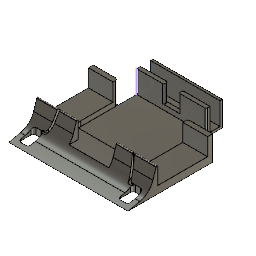
RASCUNHO_CHASSI (Autodesk Fusion 360 design; units mm, degrees)
Autodesk Fusion 360 part; units mm, degrees
sketch "Esboço1" plane through (0, 0, 0) normal (0, 0, 1) x (1, 0, 0)
  line L0 (0, 0) -> (240, 0)
  line L1 (0, 0) -> (0, 170)
  line L2 (0, 170) -> (50, 170)
  line L3 (50, 170) -> (50, 240)
  line L4 (190, 240) -> (190, 170)
  line L5 (190, 170) -> (240, 170)
  line L6 (240, 170) -> (240, 0)
  line L7 (50, 240) -> (190, 240)
  line L8 (10, 10) -> (10, 40)
  line L9 (30, 10) -> (30, 40)
  line L10 (30, 40) -> (10, 40)
  line L11 (10, 10) -> (30, 10)
  line L12 (230, 10) -> (210, 10)
  line L13 (210, 40) -> (230, 40)
  line L14 (210, 40) -> (210, 10)
  line L15 (230, 40) -> (230, 10)
  dimension "d2" = 170
  dimension "d3" = 170
  dimension "d4" = 240
  dimension "d6" = 50
  dimension "d8" = 140
  dimension "d9" = 70
  constraint coincident L0.start L1.start
  constraint horizontal L0
  constraint perpendicular L0 L1
  constraint perpendicular L1 L2
  constraint perpendicular L2 L3
  constraint perpendicular L2 L4
  constraint perpendicular L4 L5
  constraint perpendicular L2 L6
  constraint perpendicular L4 L7
  constraint perpendicular L0 L8
  constraint perpendicular L0 L9
  constraint perpendicular L9 L10
  constraint perpendicular L9 L11
  constraint perpendicular L6 L12
  constraint perpendicular L6 L13
  constraint perpendicular L12 L14
  constraint perpendicular L12 L15
  measures "d2" distance of L5.end L0.end
  measures "d3" distance of L0.start L1.end
  measures "d4" distance of L0.start L0.end
  measures "d6" distance of L4.end L5.end
  measures "d8" distance of L3.end L4.start
  measures "d9" distance of L2.end L3.end
extrude "Extrusão1" add sketch "Esboço1" along normal blind 15
fillet "Arredondamento2" radius 495 1 edges at (120, 0, 15)
sketch "Esboço5" plane through (0, 0, 0) normal (1, 0, 0) x (0, 1, 0)
  line L0 (43.5411, 8.5369) -> (60, 60)
  line L1 (60, 60) -> (60, 11)
  line L2 (43.5411, 8.5369) -> (60, 11)
  constraint vertical L1
extrude "Extrusão4" add sketch "Esboço5" along normal blind 240
fillet "Arredondamento3" radius 1.85 1 edges at (120, 60, 60)
fillet "Arredondamento4" radius 35 1 edges at (120, 43.6676, 8.9324)
delete_face "DeleteFace1" 1 faces at (80, 66.7415, 12.0246)
sketch "Esboço7" plane through (0, 0, 15) normal (0, 0, 1) x (-1, 0, 0)
  line L0 (0, -170) -> (0, -60)
  line L1 (0, -60) -> (-240, -60)
  line L2 (-240, -60) -> (-240, -170)
  line L3 (-240, -170) -> (-190, -170)
  line L4 (-190, -170) -> (-190, -240)
  line L5 (-190, -240) -> (-50, -240)
  line L6 (-50, -240) -> (-50, -170)
  line L7 (-50, -170) -> (0, -170)
  line L8 (-190, -170) -> (-190, -80)
  line L9 (-178.6152, -90) -> (-178.6152, -80)
  line L10 (-190, -80) -> (-50, -80)
  line L11 (-50, -80) -> (-50, -170)
  line L12 (-190, -170) -> (-190, -180)
  line L13 (-50, -170) -> (-50, -185)
  line L14 (-190, -185) -> (-50, -185)
  line L15 (-190, -185) -> (-190, -170)
  line L16 (-190, -170) -> (-190, -185)
  dimension "d34" = 140
  constraint coincident L3.end L4.start
  constraint perpendicular L3 L8
  constraint perpendicular L7 L9
  constraint perpendicular L8 L10
  constraint coincident L6.end L7.start
  constraint perpendicular L7 L11
  constraint coincident L4 L12.end
  constraint coincident L6 L13.end
  constraint perpendicular L7 L13
  constraint coincident L4 L14.start
  constraint perpendicular L6 L14
  measures "d34" distance of L8.end L10.end
extrude "Extrusão5" cut sketch "Esboço7" against normal blind 10 contours L4 L6 L8 L10 L11 L12 L13 L14 L15 L16
fillet "Arredondamento5" radius 15 1 edges at (190, 80, 10)
fillet "Arredondamento6" radius 15 1 edges at (50, 80, 10)
fillet "Arredondamento7" radius 5 1 edges at (230, 40, 6.7494)
fillet "Arredondamento8" radius 5 1 edges at (210, 40, 6.7494)
fillet "Arredondamento9" radius 5 1 edges at (10, 40, 6.7494)
fillet "Arredondamento10" radius 5 1 edges at (30, 40, 6.7494)
fillet "Arredondamento11" radius 5 1 edges at (10, 10, 1.2046)
fillet "Arredondamento12" radius 5 1 edges at (30, 10, 1.2046)
fillet "Arredondamento13" radius 5 1 edges at (230, 10, 1.2046)
fillet "Arredondamento14" radius 5 1 edges at (210, 10, 1.2046)
sketch "Esboço9" plane through (0, 0, 0) normal (0, 1, 0) x (1, 0, 0)
  line L0 (160, -50) -> (80, -50)
  line L1 (160, -50) -> (240, -50)
  line L2 (80, -50) -> (0, -50)
  line L3 (160, -50) -> (160, -15)
  line L4 (160, -15) -> (80, -15)
  line L5 (80, -15) -> (80, -50)
  dimension "d59" = 80
  constraint horizontal L0
  constraint parallel L0 L1
  constraint parallel L0 L2
  constraint equal L1 L2
  constraint equal L0 L2
  constraint perpendicular L0 L3
  constraint perpendicular L3 L4
  constraint perpendicular L0 L5
  measures "d59" distance of L0.start L0.end
extrude "Extrusão6" cut sketch "Esboço9" along normal blind 70
extrude "Extrusão7" cut 1 faces at (96.6667, 203.3333, 15) along direction (0, 0, -1) blind 10
sketch "Esboço10" plane through (0, 0, 5) normal (0, 0, 1) x (-1, 0, 0)
  arc A0 (-50, -95) -> (-65, -80) centre (-65, -95) ccw
  line L0 (-65, -80) -> (-175, -80)
  arc A1 (-175, -80) -> (-190, -95) centre (-175, -95) ccw
  line L1 (-190, -95) -> (-190, -170)
  line L2 (-190, -170) -> (-190, -240)
  line L3 (-190, -240) -> (-50, -240)
  line L4 (-50, -240) -> (-50, -170)
  line L5 (-50, -170) -> (-50, -95)
  line L6 (-190, -240) -> (-50, -240)
  line L7 (-190, -240) -> (-190, -235)
  line L8 (-50, -235) -> (-190, -235)
  line L9 (-50, -240) -> (-50, -235)
  constraint coincident L2.end L3.start
  constraint coincident L3.end L4.start
  constraint coincident L2 L7.end
  constraint perpendicular L3 L7
  constraint coincident L4 L8.start
  constraint perpendicular L2 L8
extrude "Extrusão8" add sketch "Esboço10" along normal blind 40 contours L2 L3 L4 L6 L7 L8 L9
sketch "Esboço15" plane through (0, 0, 0) normal (1, 0, 0) x (0, 1, 0)
extrude "Extrusão9" add 1 faces at (143.3333, 238.3333, 45) along direction (0, 0, 1) blind 5
sketch "Esboço17" plane through (0, 0, 5) normal (0, 0, 1) x (-1, 0, 0)
  line L0 (-190, -235) -> (-50, -235)
  line L1 (-50, -235) -> (-50, -170)
  line L2 (-50, -170) -> (-50, -95)
  arc A0 (-50, -95) -> (-65, -80) centre (-65, -95) ccw
  line L3 (-65, -80) -> (-175, -80)
  arc A1 (-175, -80) -> (-190, -95) centre (-175, -95) ccw
  line L4 (-190, -95) -> (-190, -170)
  line L5 (-190, -170) -> (-190, -235)
  line L6 (-50, -215) -> (-190, -215)
  line L7 (-190, -210) -> (-190, -215)
  line L8 (-50, -215) -> (-50, -210)
  line L9 (-190, -210) -> (-190, -207.0502)
  line L10 (-50, -207.0502) -> (-50, -210)
  line L11 (-190, -207.0502) -> (-50, -207.0502)
  constraint coincident L1 L6.start
  constraint perpendicular L1 L6
  constraint coincident L5 L7.start
  constraint perpendicular L6 L7
  constraint coincident L1 L8.end
  constraint coincident L5 L9.end
  constraint parallel L5 L9
  constraint coincident L1 L10.start
  constraint perpendicular L1 L11
extrude "Extrusão10" add sketch "Esboço17" along normal blind 45 contours L1 L5 L6 L7 L8 L9 L10 L11
sketch "Esboço18" plane through (50, 0, 0) normal (-1, 0, 0) x (0, -1, 0)
  line L0 (-170, 5) -> (-207.0502, 5)
  line L1 (-207.0502, 50) -> (-215, 50)
  line L2 (-215, 50) -> (-215, 5)
  line L3 (-215, 5) -> (-235, 5)
  line L4 (-235, 5) -> (-235, 50)
  line L5 (-235, 50) -> (-240, 50)
  line L6 (-240, 50) -> (-240, 0)
  line L7 (-240, 0) -> (-170, 0)
  line L8 (-170, 0) -> (-170, 5)
  line L9 (-207.0502, 5) -> (-207.0502, 50)
sketch "Esboço20" plane through (0, 0, 50) normal (0, 0, 1) x (-1, 0, 0)
  line L0 (-50, -207.0502) -> (-190, -207.0502)
  line L1 (-190, -207.0502) -> (-190, -215)
  line L2 (-190, -215) -> (-50, -215)
  line L3 (-50, -215) -> (-50, -207.0502)
  line L4 (-135.1601, -207.0502) -> (-105, -207.0502)
  line L5 (-135.1601, -207.0502) -> (-135, -215)
  line L6 (-105, -207.0502) -> (-105, -215)
  line L7 (-135, -215) -> (-105, -215)
  constraint coincident L0 L4.start
  constraint coincident L0 L4.end
  constraint coincident L2 L5.end
  constraint coincident L2 L6.end
  constraint perpendicular L6 L7
extrude "Extrusão11" cut sketch "Esboço20" against normal blind 35 contours L0 L2 L4 L5 L6 L7
sketch "Esboço22" plane through (0, 0, 15) normal (0, 0, 1) x (-1, 0, 0)
  line L0 (-160, -60) -> (-240, -60)
  line L1 (-240, -60) -> (-240, -170)
  line L2 (-240, -170) -> (-190, -170)
  line L3 (-190, -170) -> (-190, -95)
  arc A0 (-175, -80) -> (-190, -95) centre (-175, -95) ccw
  line L4 (-175, -80) -> (-65, -80)
  arc A1 (-50, -95) -> (-65, -80) centre (-65, -95) ccw
  line L5 (-50, -95) -> (-50, -170)
  line L6 (-50, -170) -> (0, -170)
  line L7 (0, -170) -> (0, -60)
  line L8 (0, -60) -> (-80, -60)
  line L9 (-80, -60) -> (-80, -41.5864)
  line L10 (-80, -41.5864) -> (-160, -41.5864)
  line L11 (-160, -41.5864) -> (-160, -60)
  line L12 (-240, -170) -> (-240, -160)
  line L13 (-190, -160) -> (-190, -170)
  line L14 (-240, -160) -> (-190, -160)
  line L15 (-50, -160) -> (0, -160)
  line L16 (0, -160) -> (0, -170)
  line L17 (0, -170) -> (-50, -170)
  line L18 (-50, -160) -> (-50, -170)
  line L19 (-240, -170) -> (-190, -170)
  constraint coincident L1.end L2.start
  constraint coincident L1 L12.end
  constraint perpendicular L2 L12
  constraint coincident L3 L13.start
  constraint coincident L2.end L3.start
  constraint perpendicular L2 L13
  constraint perpendicular L3 L14
  constraint coincident L5 L15.start
  constraint coincident L7 L15.end
  constraint perpendicular L7 L15
  constraint coincident L6.end L7.start
  constraint coincident L5.end L6.start
extrude "Extrusão12" add sketch "Esboço22" along normal blind 35 contours L1 L2 L3 L12 L13 L14 L19 | L5 L6 L7 L15 L16 L17 L18
fillet "Arredondamento15" radius 2.5 1 edges at (105, 215, 32.5)
fillet "Arredondamento16" radius 2.5 1 edges at (105, 207.0502, 32.5)
fillet "Arredondamento17" radius 5 1 edges at (50, 170, 27.5)
fillet "Arredondamento18" radius 5 1 edges at (190, 170, 27.5)
fillet "Arredondamento19" radius 2.5 1 edges at (135.1601, 207.0502, 32.5)
fillet "Arredondamento20" radius 2.5 1 edges at (135, 215, 32.5)
fillet "Arredondamento22" radius 5 1 edges at (190, 215, 27.5)
fillet "Arredondamento24" radius 2.5 1 edges at (190, 207.0502, 27.5)
delete_face "DeleteFace2" 1 faces at (186.6353, 214.725, 20)
fillet "Arredondamento28" radius 2.5 1 edges at (50, 207.0502, 27.5)
sketch "Esboço30" plane through (0, 0, 0) normal (0, 0, -1) x (1, 0, 0)
  arc A0 (30, -15) -> (25, -10) centre (25, -15) ccw
  line L0 (30, -15) -> (30, -35)
  arc A1 (25, -40) -> (30, -35) centre (25, -35) ccw
  line L1 (25, -40) -> (15, -40)
  arc A2 (10, -35) -> (15, -40) centre (15, -35) ccw
  line L2 (10, -35) -> (10, -15)
  arc A3 (15, -10) -> (10, -15) centre (15, -15) ccw
  line L3 (15, -10) -> (25, -10)
  arc A4 (215, -10) -> (210, -15) centre (215, -15) ccw
  line L4 (215, -10) -> (225, -10)
  arc A5 (230, -15) -> (225, -10) centre (225, -15) ccw
  line L5 (230, -15) -> (230, -35)
  arc A6 (225, -40) -> (230, -35) centre (225, -35) ccw
  line L6 (225, -40) -> (215, -40)
  arc A7 (210, -35) -> (215, -40) centre (215, -35) ccw
  line L7 (210, -35) -> (210, -15)
  line L8 (240, 0) -> (0, 0)
  line L9 (0, 0) -> (0, -170)
  line L10 (0, -170) -> (50, -170)
  line L11 (50, -170) -> (50, -240)
  line L12 (50, -240) -> (190, -240)
  line L13 (190, -240) -> (190, -170)
  line L14 (190, -170) -> (240, -170)
  line L15 (240, -170) -> (240, 0)
  line L16 (28.5138, -37.4693) -> (28.5355, -37.4693)
  line L17 (36, -38.0528, -10) -> (34, -38.0528, -10)
  line L18 (34, -38.0528, -10) -> (27, -38.0528, -10)
  line L19 (27, -38.0528, -10) -> (27, -41.0528, -10)
  line L20 (27, -41.0528, -10) -> (34, -41.0528, -10)
  line L21 (34, -41.0528, -10) -> (43.9831, -61.0528, -10)
  line L22 (36, -38.0528, -10) -> (48, -61.0528, -10)
  line L23 (48, -61.0528, -10) -> (43.9831, -61.0528, -10)
  line L24 (27, -41.0528, -10) -> (34, -41.0528, -10)
  line L25 (27, -38.0528, -10) -> (27, -41.0528, -10)
  line L26 (34, -38.0528, -10) -> (27, -38.0528, -10)
  line L27 (36, -38.0528, -10) -> (34, -38.0528, -10)
  line L28 (36, -38.0528, -10) -> (48, -61.0528, -10)
  line L29 (34, -41.0528, -10) -> (43.9831, -61.0528, -10)
  line L30 (48, -61.0528, -10) -> (43.9831, -61.0528, -10)
  line L31 (34, -41.0528, -10) -> (43.9831, -61.0528, -10)
  line L32 (36, -38.0528, -10) -> (48, -61.0528, -10)
  line L33 (34, -38.0528, -10) -> (27, -38.0528, -10)
  line L34 (36, -38.0528, -10) -> (34, -38.0528, -10)
  line L35 (27, -38.0528, -10) -> (27, -41.0528, -10)
  line L36 (27, -41.0528, -10) -> (34, -41.0528, -10)
  line L37 (48, -61.0528, -10) -> (43.9831, -61.0528, -10)
  line L38 (34, -41.0528, -10) -> (43.9831, -61.0528, -10)
  line L39 (36, -38.0528, -10) -> (48, -61.0528, -10)
  line L40 (34, -38.0528, -10) -> (27, -38.0528, -10)
  line L41 (36, -38.0528, -10) -> (34, -38.0528, -10)
  line L42 (27, -38.0528, -10) -> (27, -41.0528, -10)
  line L43 (27, -41.0528, -10) -> (34, -41.0528, -10)
  line L44 (48, -61.0528, -10) -> (43.9831, -61.0528, -10)
  line L45 (34, -41.0528, -10) -> (43.9831, -61.0528, -10)
  line L46 (36, -38.0528, -10) -> (48, -61.0528, -10)
  line L47 (34, -38.0528, -10) -> (27, -38.0528, -10)
  line L48 (36, -38.0528, -10) -> (34, -38.0528, -10)
  line L49 (27, -38.0528, -10) -> (27, -41.0528, -10)
  line L50 (27, -41.0528, -10) -> (34, -41.0528, -10)
  line L51 (48, -61.0528, -10) -> (43.9831, -61.0528, -10)
  line L52 (34, -41.0528, -10) -> (43.9831, -61.0528, -10)
  line L53 (36, -38.0528, -10) -> (48, -61.0528, -10)
  line L54 (34, -38.0528, -10) -> (27, -38.0528, -10)
  line L55 (36, -38.0528, -10) -> (34, -38.0528, -10)
  line L56 (27, -38.0528, -10) -> (27, -41.0528, -10)
  line L57 (27, -41.0528, -10) -> (34, -41.0528, -10)
  line L58 (48, -61.0528, -10) -> (43.9831, -61.0528, -10)
  line L59 (52, -61) -> (53, -61)
  line L60 (191.1161, -60.8778, -65) -> (195.1161, -60.8778, -65)
  line L61 (195.1161, -60.8778, -65) -> (205.6161, -40.3778, -65)
  line L62 (205.6161, -40.3778, -65) -> (212.6161, -40.3778, -65)
  line L63 (212.6161, -40.3778, -65) -> (212.6161, -37.3778, -65)
  line L64 (212.6161, -37.3778, -65) -> (203.6161, -37.3778, -65)
  line L65 (191.1161, -60.8778, -65) -> (203.6161, -37.3778, -65)
  line L66 (191.1161, -60.8778, -65) -> (203.6161, -37.3778, -65)
  line L67 (191.1161, -60.8778, -65) -> (195.1161, -60.8778, -65)
  line L68 (195.1161, -60.8778, -65) -> (205.6161, -40.3778, -65)
  line L69 (205.6161, -40.3778, -65) -> (212.6161, -40.3778, -65)
  line L70 (212.6161, -40.3778, -65) -> (212.6161, -37.3778, -65)
  line L71 (212.6161, -37.3778, -65) -> (203.6161, -37.3778, -65)
  point P0 (28.5138, -37.4693)
  dimension "d113" = 25.9422
  dimension "d114" = 22.3531
  dimension "d115" = 4.0169
  dimension "d116" = 7
  dimension "d117" = 3
  dimension "d118" = 2
  dimension "d119" = 7
  dimension "d124" = 25.9422
  dimension "d125" = 22.3531
  dimension "d126" = 4.0169
  dimension "d127" = 7
  dimension "d128" = 3
  dimension "d129" = 2
  dimension "d130" = 7
  dimension "d141" = 22.3531
  dimension "d142" = 4.0169
  dimension "d143" = 7
  dimension "d144" = 25.9422
  dimension "d145" = 22.3531
  dimension "d146" = 4.0169
  dimension "d147" = 7
  dimension "d148" = 3
  dimension "d149" = 2
  dimension "d150" = 7
  dimension "d151" = 22.3531
  dimension "d152" = 4.0169
  dimension "d153" = 7
  dimension "d154" = 25.9422
  dimension "d155" = 22.3531
  dimension "d156" = 4.0169
  dimension "d157" = 7
  dimension "d158" = 3
  dimension "d159" = 2
  dimension "d160" = 7
  dimension "d161" = 22.3531
  dimension "d162" = 4.0169
  dimension "d163" = 7
  dimension "d164" = 25.9422
  dimension "d165" = 22.3531
  dimension "d166" = 4.0169
  dimension "d167" = 7
  dimension "d168" = 3
  dimension "d169" = 2
  dimension "d170" = 7
  dimension "d171" = 22.3531
  dimension "d172" = 4.0169
  dimension "d173" = 7
  dimension "d174" = 25.9422
  dimension "d175" = 22.3531
  dimension "d176" = 4.0169
  dimension "d177" = 7
  dimension "d178" = 3
  dimension "d179" = 2
  dimension "d180" = 7
  dimension "d185" = 7
  dimension "d186" = 3
  dimension "d187" = 9
  dimension "d188" = 7
  dimension "d189" = 3
  dimension "d190" = 9
extrude "Extrusão14" cut sketch "Esboço30" against normal blind 55 contours L17 L18 L19 L20 L21 L22 L23 L24 L25 L26 L27 L28 L29 L30 L31 L32 L33 L34 L35 L36 L37 L38 L39 L40 L41 L42 L43 L44 L45 L46 L47 L48 L49 L50 L51 L52 L53 L54 L55 L56 L57 L58 in plane through (0, 0, 10) normal (0, 0, -1)
extrude "Extrusão15" add 1 faces at (41.9944, 54.3862, 10) along direction (0, 0, 1) blind 1.9
sketch "Esboço33" plane through (0, 0, 0) normal (0, 0, 1) x (1, 0, 0)
  line L0 (191.1161, -60.8778, -65) -> (203.6161, -37.3778, -65)
  line L1 (195.1161, -60.8778, -65) -> (205.6161, -40.3778, -65)
  line L2 (191.1161, -60.8778, -65) -> (195.1161, -60.8778, -65)
  line L3 (212.6161, -37.3778, -65) -> (203.6161, -37.3778, -65)
  line L4 (212.6161, -40.3778, -65) -> (212.6161, -37.3778, -65)
  line L5 (205.6161, -40.3778, -65) -> (212.6161, -40.3778, -65)
  line L6 (204.75, 40.2217, 9) -> (194.7669, 60.2217, 9)
  line L7 (202.75, 37.2217, 9) -> (190.75, 60.2217, 9)
  line L8 (204.75, 37.2217, 9) -> (211.75, 37.2217, 9)
  line L9 (211.75, 37.2217, 9) -> (211.75, 40.2217, 9)
  line L10 (211.75, 40.2217, 9) -> (204.75, 40.2217, 9)
  line L11 (202.75, 37.2217, 9) -> (204.75, 37.2217, 9)
  line L12 (190.75, 60.2217, 9) -> (194.7669, 60.2217, 9)
  dimension "d191" = 7
  dimension "d192" = 7
  dimension "d193" = 3
  dimension "d194" = 9
  dimension "d195" = 25.9422
  dimension "d196" = 4.0169
  dimension "d197" = 2
  dimension "d198" = 25.9422
  dimension "d199" = 3
  dimension "d200" = 7
  dimension "d201" = 22.3531
  dimension "d202" = 7
extrude "Extrusão16" cut sketch "Esboço33" along normal blind 55 contours L6 L7 L8 L9 L10 L11 L12 in plane through (0, 0, 9) normal (0, 0, 1)
extrude "Extrusão17" add 1 faces at (196.7556, 53.555, 9) along direction (0, 0, 1) blind 2.26
fillet "Arredondamento29" radius 6.5 1 edges at (204.75, 40.2217, 12.4788)
fillet "Arredondamento30" radius 6.5 1 edges at (34, 41.0528, 13.187)
